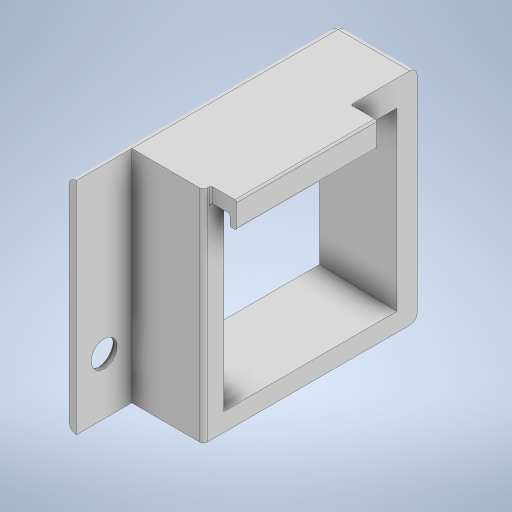
# Autodesk Inventor part: cajetinparaestructura
Saved by Autodesk Inventor 2024 (Build 280153000, 153)
## iProperties
Created: 2026-04-17
Part Number: cajetinparaestructura
Material: Genérico
Document SubType Name: Modeling
Designer: Legion
Density: 1 g/cm^3
Appearance: Valor por defecto
Author: Legion
Autodesk Inventor part; units mm, degrees
ref_plane "YZ Plane" through (0, 0, 0) normal (1, 0, 0) x (0, 1, 0)
ref_plane "XZ Plane" through (0, 0, 0) normal (0, 1, 0) x (-1, 0, 0)
ref_plane "XY Plane" through (0, 0, 0) normal (0, 0, 1) x (1, 0, 0)
sketch "Boceto1" plane through (0, 0, 0) normal (1, 0, 0) x (0, 1, 0)
  line L0 (0, 0) -> (-47.8, 0)
  line L1 (-47.8, 0) -> (-47.8, 48)
  line L2 (-47.8, 48) -> (0, 48)
  line L3 (0, 48) -> (0, 0)
  line L4 (-23.9, 48) -> (-23.9, 53)
  line L5 (-23.9, 0) -> (-23.9, -5)
  line L6 (0, 24) -> (5, 24)
  line L7 (-47.8, 24) -> (-52.8, 24)
  line L8 (5, -5) -> (-52.8, -5)
  line L9 (-52.8, -5) -> (-52.8, 53)
  line L10 (-52.8, 53) -> (5, 53)
  line L11 (5, 53) -> (5, -5)
  dimension "d0" = 47.8
  dimension "d1" = 48
  dimension "d2" = 5
  dimension "d3" = 5
  dimension "d4" = 5
  dimension "d5" = 5
  constraints: 24 end point, 4 horizontal, 4 midpoint, 4 parallel, 2 perpendicular, 2 vertical
  measures "d0" distance of L1.end L2.end
  measures "d1" distance of L0.end L1.end
  measures "d2" distance of L4.start L4.end
  measures "d3" distance of L5.start L5.end
  measures "d4" distance of L6.start L6.end
  measures "d5" distance of L7.start L7.end
extrude "Extrusión1" add sketch "Boceto1" along normal blind 21.5 contours L3 L6 L11 L8 L5 L0 | L5 L8 L9 L7 L1 L0 | L3 L2 L4 L10 L11 L6 | L7 L9 L10 L4 L2 L1
sketch "Boceto2" plane through (0, 0, 0) normal (-1, 0, 0) x (0, 0, 1)
  line L0 (53, 5) -> (53, -52.8) projected
  line L1 (53, 5) -> (68, 5)
  line L2 (68, 5) -> (68, -52.8)
  line L3 (68, -52.8) -> (53, -52.8)
  line L4 (53, -52.8) -> (53, 5)
  point P0 (0, 0)
  dimension "d8" = 15
  constraints: 8 end point, 2 parallel, 1 horizontal, 1 perpendicular
  measures "d8" distance of L2.end L3.end
extrude "Extrusión2" add sketch "Boceto2" against normal blind 2
sketch "Boceto3" plane through (21.5, 0, 0) normal (1, 0, 0) x (0, 0, -1)
  line L0 (-51, 5) -> (-13, 5)
  line L1 (-13, 3) -> (-51, 3)
  line L2 (-51, 5) -> (-51, 3)
  line L3 (-13, 5) -> (-13, 3)
  constraints: 8 end point, 2 perpendicular, 1 horizontal, 1 parallel
extrude "Extrusión3" add sketch "Boceto3" along normal blind 7
sketch "Boceto4" plane through (21.5, 3, 13) normal (0, -1, 0) x (1, 0, 0)
  line L0 (0, 38) -> (7, 38) projected
  line L1 (0, 0) -> (7, 0) projected
  line L2 (7, 38) -> (5.2, 38)
  line L3 (5.2, 38) -> (5.2, 0)
  line L4 (5.2, 0) -> (7, 0)
  line L5 (7, 0) -> (7, 38)
  point P0 (-21.5, -13)
  point P1 (7, 0)
  dimension "d16" = 1.8
  constraints: 8 end point, 2 parallel, 1 horizontal, 1 perpendicular, 1 point on line
  measures "d16" distance of L4.end L3.end
extrude "Extrusión4" add sketch "Boceto4" along normal blind 3
sketch "Boceto5" plane through (0, 0, 0) normal (-1, 0, 0) x (0, 0, 1)
  line L0 (60.5, 5) -> (60.5, -37.5)
  dimension "d19" = 42.5
  constraints: 2 end point, 1 coincident, 1 vertical
  measures "d19" distance of L0.start L0.end
hole "Agujero1" at (0, -37.5, 60.5) direction (1, 0, 0) diameter 7 depth 2 countersink diameter 9 countersink angle 90
fillet "Empalme3" radius 0.5 2 edges at (28.5, 0, 32) (26.7, 0, 32)
sketch "Boceto6" plane through (21.5, 0, 0) normal (1, 0, 0) x (0, 0, -1)
  line L0 (-48, -47.8) -> (-48, 0) projected
  line L1 (0, -47.8) -> (-48, -47.8) projected
  line L2 (-48, 0) -> (-47.5, 0)
  line L3 (-47.5, 0) -> (-47.5, -47.8)
  line L4 (-47.5, -47.8) -> (-48, -47.8)
  line L5 (-48, -47.8) -> (-48, 0)
  line L6 (-48, 0) -> (0, 0) projected
  line L7 (0, -47.8) -> (-0.5, -47.8)
  line L8 (-0.5, -47.8) -> (-0.5, 0)
  line L9 (-0.5, 0) -> (0, 0)
  line L10 (0, 0) -> (0, -47.8)
  dimension "d30" = 0.5
  dimension "d31" = 0.5
  constraints: 16 end point, 4 parallel, 2 horizontal, 2 perpendicular, 2 point on line
  measures "d30" distance of L3.end L4.end
  measures "d31" distance of L8.end L9.end
extrude "Extrusión5" add sketch "Boceto6" against normal blind 21.5 contours L0 L2 L3 L1 | L8 L6 L10 L1
chamfer "Chaflán1" distance 0.5 distance2 21.5 2 edges at (0, -23.9, 0.5) (0, -23.9, 47.5) measured on face at (0, -9.3443, 58.8475)
fillet "Empalme4" radius 1 1 edges at (21.5, -23.9, 53)
sketch "Boceto7" plane through (0, 5, -5) normal (0, 1, 0) x (1, 0, 0)
  arc A0 (20.5, -58) -> (21.5, -57) centre (20.5, -57) ccw projected
  line L0 (21.5, -56) -> (21.5, -57) projected
  line L1 (21.5, -56) -> (28.5, -56) projected
  line L2 (28.5, -18) -> (28.5, -56) projected
  line L3 (21.5, -18) -> (28.5, -18) projected
  line L4 (21.5, 0) -> (21.5, -18) projected
  line L5 (0, 0) -> (21.5, 0) projected
  line L6 (0, 0) -> (0, -73) projected
  line L7 (0, -73) -> (2, -73) projected
  line L8 (2, -58) -> (2, -73) projected
  line L9 (2, -58) -> (20.5, -58) projected
  point P0 (0, -5)
extrude "Extrusión6" add sketch "Boceto7" along normal blind 2
fillet "Empalme6" radius 2 5 edges at (0, 7, 31.5) (10.75, 7, -5) (0, -22.9, -5) (10.75, -52.8, -5) (0, -52.8, 31.5)
fillet "Empalme7" radius 0.5 5 edges at (28.5, 7, 32) (21.5, 3, 32) (26.7, 3, 32) (21.5, 5, 13) (21.5, 5, 51)
